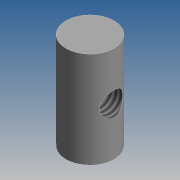
# Autodesk Inventor part: P109
Saved by Autodesk Inventor 2019 (Build 230136000, 136)
## iProperties
Created: 2016-10-19
Part Number: P109
Material: Acier / Stahl
Document SubType Name: Modeling
Designer: serge.amoos
Density: 7.85 g/cm^3
Appearance: Par défaut
Description: Ecrou
Author: serge.amoos
Autodesk Inventor part; units mm, degrees
ref_plane "XZ Plane" through (0, 0, 0) normal (0, 1, 0) x (-1, 0, 0)
ref_plane "XY Plane" through (0, 0, 0) normal (0, 0, 1) x (1, 0, 0)
sketch "Sketch1" plane through (0, 0, 0) normal (0, 0, 1) x (1, 0, 0)
  circle A0 centre (0, 0) radius 2.5
  dimension "d0" = 5
  constraints: 1 centre point, 1 coincident
  measures "d0" diameter of A0
extrude "Extrusion1" add sketch "Sketch1" along normal mid plane 10
ref_plane "Work Plane1" through (3, 0, 0) normal (1, 0, 0) x (0, 1, 0)
sketch "Sketch3" plane through (3, 0, 0) normal (1, 0, 0) x (0, 1, 0)
  point P0 (0, 0)
hole "Hole1" at (3, 0, 0) direction (-1, 0, 0) diameter 2.459 end through all thread size "M3x0.5" class "6H" standard "ISO Metric profile"
body "Solid1"
